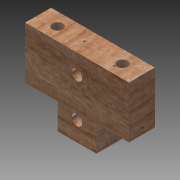
# Autodesk Inventor part: X_Bottem_MotorSide_V3
Saved by Autodesk Inventor 2014 (Build 180170000, 170)
## iProperties
Created: 2013-12-16
Part Number: X_Bottem_MotorSide_V3
Material: Birch
Document SubType Name: Modeling
Designer: Bram
Density: 0.512 g/cm^3
Appearance: Birch - Natural Medium Gloss
Author: Bram
Autodesk Inventor part; units mm, degrees
ref_plane "YZ Plane" through (0, 0, 0) normal (1, 0, 0) x (0, 1, 0)
ref_plane "XZ Plane" through (0, 0, 0) normal (0, 1, 0) x (-1, 0, 0)
ref_plane "XY Plane" through (0, 0, 0) normal (0, 0, 1) x (1, 0, 0)
sketch "Sketch1" plane through (0, 0, 0) normal (0, 1, 0) x (-1, 0, 0)
  line L0 (0, 0) -> (80, 0)
  line L1 (80, 0) -> (80, 60)
  line L2 (80, 60) -> (0, 60)
  line L3 (0, 60) -> (0, 0)
  circle A0 centre (40, 45) radius 4
  circle A1 centre (40, 15) radius 4
  dimension "d0" = 80
  dimension "d1" = 60
  dimension "d4" = 8
  dimension "d5" = 8
  constraints: 8 end point, 2 centre point, 2 parallel, 1 horizontal, 1 perpendicular
  measures "d0" distance of L2.end L1.end
  measures "d1" distance of L1.end L0.end
  measures "d4" diameter of A0
  measures "d5" diameter of A1
extrude "Extrusion1" add sketch "Sketch1" along normal blind 20
sketch "Sketch2" plane through (-80, 0, 60) normal (0, 0, 1) x (1, 0, 0)
  circle A0 centre (15, 10) radius 4
  circle A1 centre (65, 10) radius 4
  dimension "d10" = 8
  dimension "d11" = 8
  constraints: 2 centre point
  measures "d10" diameter of A0
  measures "d11" diameter of A1
extrude "Extrusion2" cut sketch "Sketch2" against normal blind 60
sketch "Sketch3" plane through (0, 20, 0) normal (0, 1, 0) x (1, 0, 0)
  line L0 (0, 0) -> (-80, 0) projected
  line L1 (-80, 0) -> (-80, -60) projected
  line L2 (0, -60) -> (0, 0) projected
  line L3 (-40, 0) -> (-25, 0)
  line L4 (-40, 0) -> (-55, 0)
  line L5 (-80, -60) -> (-80, -20)
  line L6 (-80, -20) -> (-55, -20)
  line L7 (-55, -20) -> (-55, 0)
  line L8 (0, -20) -> (-25, -20)
  line L9 (-25, -20) -> (-25, 0)
  dimension "d14" = 15
  dimension "d15" = 15
  dimension "d16" = 40
  constraints: 14 end point, 4 point on line, 3 perpendicular, 1 midpoint, 1 parallel
  measures "d14" distance of L3.start L3.end
  measures "d15" distance of L3.start L4.end
  measures "d16" distance of L1.end L5.end
extrude "Extrusion3" cut sketch "Sketch3" against normal blind 60
body "Solid1"
